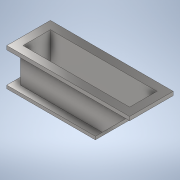
# Autodesk Inventor part: Корпус
Saved by Autodesk Inventor 2022.1 (Build 261234020, 234B)
## iProperties
Created: 2021-12-02
Part Number: Корпус
Material: Сталь, углеродистая
Document SubType Name: Modeling
Designer: Алексанян Г.
Density: 7.85 g/cm^3
Appearance: С умеренной полировкой
Author: Алексанян Г.
Autodesk Inventor part; units mm, degrees
ref_plane "YZ Plane" through (0, 0, 0) normal (1, 0, 0) x (0, 1, 0)
ref_plane "XZ Plane" through (0, 0, 0) normal (0, 1, 0) x (-1, 0, 0)
ref_plane "XY Plane" through (0, 0, 0) normal (0, 0, 1) x (1, 0, 0)
sketch "Эскиз1" plane through (0, 0, 0) normal (0, 1, 0) x (-1, 0, 0)
  line L0 (493, -175) -> (-493, -175)
  line L1 (-493, -175) -> (-493, 175)
  line L2 (-493, 175) -> (493, 175)
  line L3 (493, 175) -> (493, -175)
  line L4 (493, -175) -> (-493, 175) construction
  line L5 (-493, -175) -> (493, 175) construction
  point P0 (0, 0)
  dimension "d0" = 986
  dimension "d1" = 350
  constraints: 12 end point, 2 midpoint, 2 parallel, 1 horizontal, 1 perpendicular
  measures "d0" distance of L0.start L0.end
  measures "d1" distance of L2.end L0.start
extrude "Выдавливание1" add sketch "Эскиз1" against normal blind 300
sketch "Эскиз2" plane through (0, -300, 0) normal (0, -1, 0) x (1, 0, 0)
  line L0 (493, 175) -> (-493, 175) projected
  line L1 (-493, 175) -> (-493, -175) projected
  line L2 (-493, -175) -> (493, -175) projected
  line L3 (493, -175) -> (493, 175) projected
  line L4 (-438, 120) -> (438, 120)
  line L5 (438, 120) -> (438, -120)
  line L6 (438, -120) -> (-438, -120)
  line L7 (-438, -120) -> (-438, 120)
  point P0 (0, 0)
  dimension "d4" = 55
  constraints: 8 end point, 3 other
  measures "d4" distance between parallel lines of L0 L4
extrude "Выдавливание2" cut sketch "Эскиз2" against normal blind 270
sketch "Эскиз4" plane through (-493, 0, 175) normal (0, 0, 1) x (1, 0, 0)
  line L0 (0, 0) -> (986, 0) projected
  line L1 (986, 0) -> (711, -275)
  line L2 (986, 0) -> (1374.9087, 0) construction
  line L3 (931, -300) -> (55, -300) projected
  line L4 (931, -55) -> (931, -300)
  line L5 (931, -300) -> (931, -30) projected
  line L6 (711, -275) -> (711, -300)
  line L7 (711, -300) -> (931, -300)
  point P0 (493, 0)
  dimension "d10" = 135
  dimension "d13" = 25
  constraints: 10 end point, 2 horizontal, 2 point on line, 1 equal length, 1 vertical
  measures "d10" angle of L1 L2
  measures "d13" distance from line of L3 L1.end
extrude "Выдавливание3" cut sketch "Эскиз4" against normal through all
sketch "Эскиз5" plane through (0, -300, 0) normal (0, -1, 0) x (1, 0, 0)
  line L0 (-493, -175) -> (-493, 175) construction
  line L1 (493, -175) -> (-493, -175) construction
  line L2 (493, 175) -> (493, -175) construction
  line L3 (-493, 175) -> (493, 175) construction
  line L4 (438, 120) -> (-438, 120) construction
  line L5 (438, -120) -> (438, 120) construction
  line L6 (-438, -120) -> (438, -120) construction
  line L7 (-438, 120) -> (-438, -120) construction
  line L8 (-493, 175) -> (493, 175) projected
  line L9 (218, 175) -> (-493, 175)
  line L10 (-493, -175) -> (-493, 175) projected
  line L11 (-493, 175) -> (-493, -175)
  line L12 (-493, -175) -> (218, -175)
  line L13 (493, -175) -> (-493, -175) projected
  line L14 (218, 175) -> (218, -175)
  point P0 (0, 0)
  point P1 (218, 120)
  constraints: 8 end point, 3 point on line, 2 collinear, 1 perpendicular
extrude "Выдавливание5" add sketch "Эскиз5" against normal blind 25
shell "Оболочка1" thickness 10 removed faces 1 at (-164.3333, 0, -58.3333)
sketch "Эскиз6" plane through (-483, -20, 165) normal (0, 1, 0) x (1, 0, 0)
  line L0 (0, 330) -> (0, 0) projected
  line L1 (0, 0) -> (966, 0) projected
  line L2 (966, 0) -> (966, 330) projected
  line L3 (966, 330) -> (0, 330) projected
  line L4 (911, 55) -> (55, 55) projected
  line L5 (55, 55) -> (55, 275) projected
  line L6 (55, 275) -> (911, 275) projected
  line L7 (911, 275) -> (911, 55) projected
  point P0 (483, 165)
extrude "Выдавливание6" add sketch "Эскиз6" along normal up to surface (20 mm away)
sketch "Эскиз7" plane through (-483, -290, -165) normal (0, 1, 0) x (1, 0, 0)
  line L0 (691, 0) -> (691, -330) projected
  line L1 (0, 0) -> (691, 0) projected
  line L2 (0, -330) -> (0, 0) projected
  line L3 (691, -330) -> (0, -330) projected
  point P0 (483, -165)
extrude "Выдавливание7" add sketch "Эскиз7" along normal up to surface (5 mm away)
